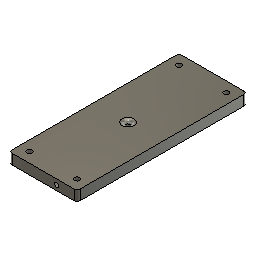
Down Table v5 (Autodesk Fusion 360 design; units mm, degrees)
Autodesk Fusion 360 part; units mm, degrees
sketch "Sketch1" plane through (0, 0, 0) normal (0, 1, 0) x (1, 0, 0)
  line L0 (0, 130) -> (0, -122.2085) construction
  line L1 (-100, 0) -> (125, 0) construction
  line L2 (40, 100) -> (-40, 100)
  line L3 (-40, 100) -> (-40, -100)
  line L4 (-40, -100) -> (40, -100)
  line L5 (40, -100) -> (40, 100)
  line L6 (40, 100) -> (-40, -100) construction
  line L7 (-40, 100) -> (40, -100) construction
  circle A0 centre (-28, -88) radius 3
  circle A1 centre (0, 0) radius 3
  circle A2 centre (-28, 88) radius 3
  circle A3 centre (28, 88) radius 3
  circle A4 centre (28, -88) radius 3
  dimension "d1" = 80
  dimension "d2" = 200
  dimension "d3" = 6
  dimension "d4" = 6
  dimension "d5" = 12
  dimension "d6" = 12
  constraint vertical L0
  constraint horizontal L1
  constraint horizontal L2
  constraint perpendicular L2 L3
  constraint parallel L2 L4
  constraint parallel L3 L5
  constraint coincident L6 A1.centre
  constraint coincident L7 A1.centre
  constraint coincident A1.centre origin
  constraint symmetric L1 A0 A2
  constraint symmetric L0 A0 A4
  constraint symmetric L0 A2 A3
  measures "d1" distance of L3.end L4.end
  measures "d2" distance of L2.end L3.end
  measures "d3" diameter of A0
  measures "d4" diameter of A1
  measures "d5" distance of L4 A0.centre
  measures "d6" distance of L3 A0.centre
extrude "Extrude1" add sketch "Sketch1" along normal blind 12
fillet "Fillet1" radius 4 1 edges at (-2.797, 12, -1.0848)
fillet "Fillet2" radius 3.5 4 edges at (40, 6, -100) (-40, 6, -100) (-40, 6, 100) (40, 6, 100)
sketch "Sketch2" plane through (0, 0, 100) normal (0, 0, 1) x (1, 0, 0)
  line L0 (36.5, 0) -> (36.5, 12)
  line L1 (36.5, 12) -> (-36.5, 12)
  line L2 (-36.5, 12) -> (-36.5, 0)
  line L3 (-36.5, 0) -> (36.5, 0)
  line L4 (0, 12) -> (0, 0) construction
  line L5 (7, 12) -> (7, 0) construction
  line L6 (7, 12) -> (-7, 12) construction
  line L7 (25, 12) -> (31, 12) construction
  line L8 (25, 12) -> (25, 0) construction
  line L9 (25, 0) -> (7, 12) construction
  line L10 (7, 0) -> (25, 12) construction
  circle A0 centre (16, 6) radius 2.5
  dimension "d13" = 7
  dimension "d14" = 14
  dimension "d15" = 6
  dimension "d16" = 5
  constraint midpoint L1 L4.start
  constraint coincident L4.end origin
  constraint coincident L1 L5.start
  constraint coincident L3 L5.end
  constraint perpendicular L3 L5
  constraint coincident L7.start L8.start
  constraint coincident L3 L8.end
  constraint perpendicular L3 L8
  constraint midpoint L9 A0.centre
  measures "d13" distance of L4 L5
  measures "d14" distance of L5.start L6.end
  measures "d15" distance of L7.start L7.end
  measures "d16" diameter of A0
extrude "Extrude2" cut sketch "Sketch2" against normal blind 200 contours A0
equation "d6 = d5"
equation "d13 = d14 / 2"
